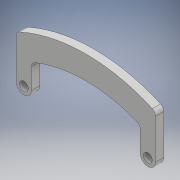
# Autodesk Inventor part: Light Sensor Cover
Saved by Autodesk Inventor 2017 (Build 210142000, 142)
## iProperties
Created: 2017-03-23
Part Number: Light Sensor Cover
Material: Generic
Document SubType Name: Modeling
Designer: yella
Density: 1 g/cm^3
Appearance: Default
Author: yella
Autodesk Inventor part; units mm, degrees
ref_plane "YZ Plane" through (0, 0, 0) normal (1, 0, 0) x (0, 1, 0)
ref_plane "XZ Plane" through (0, 0, 0) normal (0, 1, 0) x (-1, 0, 0)
ref_plane "XY Plane" through (0, 0, 0) normal (0, 0, 1) x (1, 0, 0)
sketch "Sketch1" plane through (0, 0, 0) normal (0, 1, 0) x (-1, 0, 0)
  circle A0 centre (22.6343, 38) radius 1.6
  circle A1 centre (-22.6343, 38) radius 1.6
  arc A2 (19.8343, 38) -> (25.4343, 38) centre (22.6343, 38) ccw
  arc A3 (-25.4343, 38) -> (-19.8343, 38) centre (-22.6343, 38) ccw
  line L0 (-25.4343, 38) -> (-25.4343, 52.5079)
  line L1 (25.4343, 38) -> (25.4343, 52.5079)
  arc A4 (18.5623, 47.502) -> (-18.5623, 47.502) centre (0, 0) ccw
  line L2 (19.8343, 45.6392) -> (19.8343, 38)
  line L3 (-19.8343, 45.6392) -> (-19.8343, 38)
  arc A5 (24.2494, 54.3343) -> (-24.2494, 54.3343) centre (0, 0) ccw
  arc A6 (25.4343, 52.5079) -> (24.2494, 54.3343) centre (23.4343, 52.5079) ccw
  arc A7 (19.8343, 45.6392) -> (18.5623, 47.502) centre (17.8343, 45.6392) ccw
  arc A8 (-24.2494, 54.3343) -> (-25.4343, 52.5079) centre (-23.4343, 52.5079) ccw
  arc A9 (-18.5623, 47.502) -> (-19.8343, 45.6392) centre (-17.8343, 45.6392) ccw
  point P0 (-25.4343, 53.7898)
  point P1 (25.4343, 53.7898)
  point P2 (19.8343, 46.9851)
  point P3 (-19.8343, 46.9851)
  dimension "d3" = 3.2
  dimension "d4" = 2.8
  dimension "d5" = 2.8
  dimension "d7" = 2
  constraints: 20 point on circle, 10 centre point, 8 end point, 8 tangent, 4 point on line, 3 coincident, 3 equal radius, 2 parallel, 2 vertical
  measures "d3" diameter of A0
  measures "d4" radius of A2
  measures "d5" radius of A3
  measures "d7" radius of A6
extrude "Extrusion1" add sketch "Sketch1" along normal blind 3
body "Solid1"
